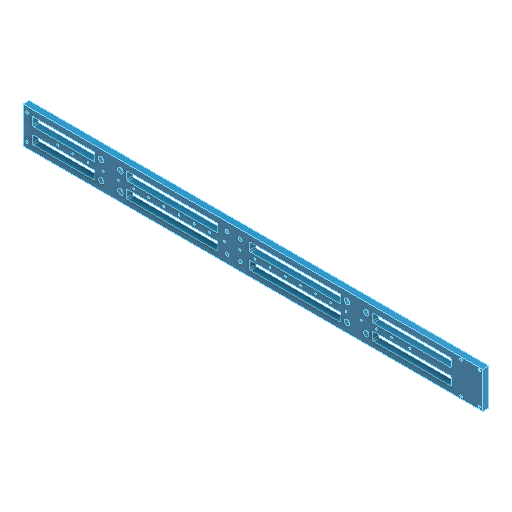
# Autodesk Inventor part: z_plate
Saved by Autodesk Inventor 2026.1 (Build 301233000, 233)
## iProperties
Created: 2025-09-27
Part Number: z_plate
Material: Aluminum 6061
Document SubType Name: Modeling
Designer: drago
Density: 2.7 g/cm^3
Appearance: Sky Blue Dark
Author: drago
Autodesk Inventor part; units mm, degrees
ref_plane "YZ Plane" through (0, 0, 0) normal (1, 0, 0) x (0, 1, 0)
ref_plane "XZ Plane" through (0, 0, 0) normal (0, 1, 0) x (-1, 0, 0)
ref_plane "XY Plane" through (0, 0, 0) normal (0, 0, 1) x (1, 0, 0)
sketch "Sketch1" plane through (0, 0, 0) normal (0, 0, 1) x (1, 0, 0)
  line L0 (-228.5, 30) -> (228.5, 30)
  line L1 (228.5, 30) -> (228.5, -30)
  line L2 (228.5, -30) -> (-228.5, -30)
  line L3 (-228.5, -30) -> (-228.5, 30)
  line L4 (0, 30) -> (0, -30) construction
  line L5 (-202.5, 30) -> (-202.5, -30) construction
  line L6 (202.5, 30) -> (202.5, -30) construction
  line L7 (-176.5, 30) -> (-176.5, -30)
  line L8 (176.5, 30) -> (176.5, -30)
  line L9 (228.5, 0) -> (-228.5, 0) construction
  line L10 (-26, 30) -> (-26, -30)
  line L11 (26, 30) -> (26, -30)
  line L12 (-228.5, 30) -> (-347, 30)
  line L13 (-347, 30) -> (-347, -30)
  line L14 (-347, -30) -> (-228.5, -30)
  line L15 (-332, 30) -> (-332, -30)
  line L16 (228.5, 30) -> (410.5, 30)
  line L17 (410.5, 30) -> (410.5, -30)
  line L18 (410.5, -30) -> (228.5, -30)
  line L19 (358.5, 30) -> (358.5, -30)
  line L20 (332, 30) -> (332, -30) construction
  line L21 (-332, 20) -> (-228.5, 20)
  line L22 (-176.5, 20) -> (-26, 20)
  line L23 (26, 20) -> (176.5, 20)
  line L24 (228.5, 20) -> (358.5, 20)
  line L25 (-332, -20) -> (-228.5, -20)
  line L26 (-176.5, -20) -> (-26, -20)
  line L27 (26, -20) -> (176.5, -20)
  line L28 (228.5, -20) -> (358.5, -20)
  line L29 (-332, 6) -> (-228.5, 6)
  line L30 (-176.5, 6) -> (-26, 6)
  line L31 (26, 6) -> (176.5, 6)
  line L32 (228.5, 6) -> (358.5, 6)
  line L33 (-332, -6) -> (-228.5, -6)
  line L34 (-176.5, -6) -> (-26, -6)
  line L35 (26, -6) -> (176.5, -6)
  line L36 (228.5, -6) -> (358.5, -6)
  line L37 (-228.5, 0) -> (-347, 0) construction
  line L38 (228.5, 0) -> (410.5, 0) construction
  line L39 (384.5, 30) -> (384.5, -30) construction
  line L40 (-339.5, 30) -> (-339.5, -30) construction
  circle A0 centre (404.5, 26) radius 2.1
  circle A1 centre (374.5, 26) radius 2.1
  circle A2 centre (374.5, -26) radius 2.1
  circle A3 centre (404.5, -26) radius 2.1
  circle A4 centre (-340.5, 21) radius 2.1
  circle A5 centre (-340.5, -21) radius 2.1
  line L41 (-300, 6) -> (-300, -6) construction
  line L42 (300, 6) -> (300, -6) construction
  circle A6 centre (-290, 0) radius 1.6
  point P0 (0, 0)
  point P1 (0, 0)
  point P2 (-218.5, 15)
  point P3 (-186.5, 15)
  point P4 (-186.5, -15)
  point P5 (-218.5, -15)
  point P6 (186.5, 15)
  point P7 (218.5, 15)
  point P8 (218.5, -15)
  point P9 (186.5, -15)
  point P10 (-11, 16)
  point P11 (11, 16)
  point P12 (11, -16)
  point P13 (-11, -16)
  point P14 (-290, 0)
  point P15 (-265, 0)
  point P16 (-240, 0)
  point P17 (-215, 0)
  point P18 (-190, 0)
  point P19 (-165, 0)
  point P20 (-140, 0)
  point P21 (-115, 0)
  point P22 (-90, 0)
  point P23 (-65, 0)
  point P24 (-40, 0)
  point P25 (-15, 0)
  point P26 (10, 0)
  point P27 (35, 0)
  point P28 (60, 0)
  point P29 (85, 0)
  point P30 (110, 0)
  point P31 (135, 0)
  point P32 (160, 0)
  point P33 (185, 0)
  point P34 (210, 0)
  point P35 (235, 0)
  point P36 (260, 0)
  point P37 (290, 0)
  dimension "d39" = 405
  dimension "d42" = 52
  dimension "d43" = 30
  dimension "d44" = 32
  dimension "d45" = 32
  dimension "d46" = 30
  dimension "d52" = 52
  dimension "d53" = 15
  dimension "d54" = 60
  dimension "d56" = 52
  dimension "d57" = 78.5
  dimension "d60" = 10
  dimension "d61" = 10
  dimension "d62" = 12
  dimension "d74" = 4.2
  dimension "d78" = 4
  dimension "d79" = 6
  dimension "d80" = 30
  dimension "d81" = 4
  dimension "d82" = 4.2
  dimension "d83" = 6.5
  dimension "d84" = 9
  dimension "d93" = 32
  dimension "d94" = 22
  dimension "d131" = 600
  dimension "d132" = 10
  dimension "d135" = 25
  dimension "d140" = 10
  dimension "d141" = 3.2
  dimension "d142" = 32
  dimension "d143" = 32
  constraints: 82 end point, 60 point on line, 17 perpendicular, 12 symmetric about line, 8 collinear, 8 vertical, 7 centre point, 5 midpoint, 4 equal radius, 4 horizontal, 2 coincident, 2 parallel, 53 other
  measures "d39" distance between parallel lines of L6 L5
  measures "d42" distance between parallel lines of L11 L10
  measures "d43" distance of point (-186.5, -15) point (-186.5, 15)
  measures "d44" distance of point (-186.5, -15) point (-218.5, -15)
  measures "d45" distance of point (218.5, -15) point (186.5, -15)
  measures "d46" distance of point (218.5, -15) point (218.5, 15)
  measures "d52" distance between parallel lines of L7 L3
  measures "d53" distance between parallel lines of L15 L13
  measures "d54" distance of L16.end L17.end
  measures "d56" distance between parallel lines of L17 L19
  measures "d57" distance between parallel lines of L17 L20
  measures "d60" distance between parallel lines of L12 L21
  measures "d61" distance between parallel lines of L14 L25
  measures "d62" distance between parallel lines of L33 L29
  measures "d74" diameter of A0
  measures "d78" distance from line of L16 A0.centre
  measures "d79" distance from line of L17 A0.centre
  measures "d80" distance of A0.centre A1.centre
  measures "d81" distance from line of L16 A1.centre
  measures "d82" diameter of A4
  measures "d83" distance from line of L13 A4.centre
  measures "d84" distance from line of L12 A4.centre
  measures "d93" distance of point (11, -16) point (11, 16)
  measures "d94" distance of point (11, 16) point (-11, 16)
  measures "d131" distance between parallel lines of L41 L42
  measures "d132" distance from line of L41 point (-290, 0)
  measures "d135" distance of point (-290, 0) point (-265, 0)
  measures "d140" distance from line of L42 point (290, 0)
  measures "d141" diameter of A6
  measures "d142" distance between parallel lines of L41 L15
  measures "d143" distance between parallel lines of L42 L20
extrude "Extrusion2" add sketch "Sketch1" against normal blind 10 contours L0 L7 L2 L3 | L3 L21 L15 L12 | L0 L10 L22 L7 | L15 L14 L13 L12 | L0 L11 L2 L10 | L3 L33 L15 L29 | L0 L8 L23 L11 | L30 L10 L34 L7 | L0 L1 L2 L8 | L3 L14 L15 L25 | L16 L19 L24 L1 | L31 L8 L35 L11 | L26 L10 L2 L7 | L16 L17 L18 L19 | L32 L19 L36 L1 | L27 L8 L2 L11 | L28 L19 L18 L1 | A0 | A1 | A2 | A3 | A4 | A5 | A6
hole "Hole2" at (-218.5, 15, 0) at (-186.5, 15, 0) at (-186.5, -15, 0) at (-218.5, -15, 0) at (186.5, 15, 0) at (218.5, 15, 0) at (218.5, -15, 0) at (186.5, -15, 0) direction (0, 0, -1) diameter 5.2 end through all counterbore diameter 9 counterbore depth 5
hole "Hole3" at (-340.5, 21, 0) at (-340.5, -21, 0) at (374.5, 26, 0) at (404.5, 26, 0) at (404.5, -26, 0) at (374.5, -26, 0) direction (0, 0, -1) diameter 4.2 end through all
hole "Hole4" at (-11, 16, 0) at (11, 16, 0) at (11, -16, 0) at (-11, -16, 0) direction (0, 0, -1) diameter 3.2 end through all counterbore diameter 6 counterbore depth 5
hole "Hole6" at (-290, 0, 0) at (-265, 0, 0) at (-240, 0, 0) at (-215, 0, 0) at (-190, 0, 0) at (-165, 0, 0) at (-140, 0, 0) at (-115, 0, 0) at (-90, 0, 0) at (-65, 0, 0) at (-40, 0, 0) at (-15, 0, 0) at (10, 0, 0) at (35, 0, 0) at (60, 0, 0) at (85, 0, 0) at (110, 0, 0) at (135, 0, 0) at (160, 0, 0) at (185, 0, 0) at (210, 0, 0) at (235, 0, 0) at (260, 0, 0) at (290, 0, 0) direction (0, 0, -1) diameter 3.2 depth 20
fillet "Fillet1" radius 2 32 edges at (-332, 6, -5) (-332, -20, -5) (-176.5, 6, -5) (-176.5, -20, -5) (26, 6, -5) (26, -20, -5) (228.5, 6, -5) (228.5, -20, -5) (228.5, 20, -5) (228.5, -6, -5) (26, 20, -5) (26, -6, -5) (-176.5, -6, -5) (-176.5, 20, -5) (-332, 20, -5) (-332, -6, -5) (-228.5, 20, -5) (-228.5, -6, -5) (-26, 20, -5) (-26, -6, -5) (176.5, 20, -5) (176.5, -6, -5) (358.5, 20, -5) (358.5, -6, -5) (358.5, 6, -5) (358.5, -20, -5) (176.5, 6, -5) (176.5, -20, -5) (-26, 6, -5) (-26, -20, -5) (-228.5, 6, -5) (-228.5, -20, -5)
equation "\"d39\" = dist_rails"
equation "\"d42\" = bracket_width"
equation "\"dist_rails\" = 405"
equation "\"bracket_width\" = 52"
body "Solid2"
